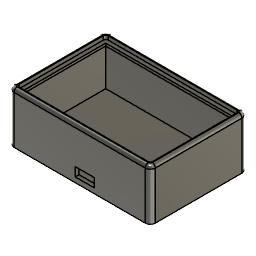
full macropad (Autodesk Fusion 360 archive; units mm, degrees)
design "macro  pad back up"
part number: 2026-03-02-20-18-01-878
Autodesk Fusion 360 part; units mm, degrees
sketch "Sketch1" plane through (0, 0, 0) normal (0, 0, 1) x (1, 0, 0)
  line L0 (-52.5, 35) -> (52.5, 35)
  line L1 (52.5, 35) -> (52.5, -35)
  line L2 (52.5, -35) -> (-52.5, -35)
  line L3 (-52.5, -35) -> (-52.5, 35)
  line L4 (-55.5, 38) -> (55.5, 38)
  line L5 (55.5, 38) -> (55.5, -38)
  line L6 (55.5, -38) -> (-55.5, -38)
  line L7 (-55.5, -38) -> (-55.5, 38)
  dimension "d1" = 105
  dimension "d2" = 70
  dimension "d3" = 35
  dimension "d4" = 52.5
  dimension "d5" = 111
  dimension "d6" = 76
  dimension "d7" = 3
  dimension "d8" = 3
  constraint horizontal L0
  constraint vertical L1
  constraint horizontal L2
  constraint vertical L3
  constraint horizontal L4
  constraint vertical L5
  constraint horizontal L6
  constraint vertical L7
  measures "d1" distance of L0.start L0.end
  measures "d2" distance of L0.start L2.end
  measures "d3" distance of origin L0
  measures "d4" distance of origin L3
  measures "d5" distance of L4.start L4.end
  measures "d6" distance of L4.start L6.end
  measures "d7" distance of L0 L4
  measures "d8" distance of L3 L7
extrude "Extrude1" add sketch "Sketch1" along normal blind 3 contours L0 L1 L2 L3 makes body 1
extrude "Extrude2" add sketch "Sketch1" along normal blind 40 bodies 1
fillet "Fillet1" radius 4 4 edges at (55.5, -38, 20) (55.5, 38, 20) (-55.5, -38, 20) (-55.5, 38, 20) on bodies 1
fillet "Fillet2" radius 2.5 8 edges at (54.3284, -36.8284, 40) (55.5, 0, 40) (54.3284, 36.8284, 40) (0, 38, 40) (-54.3284, 36.8284, 40) (-55.5, 0, 40) (-54.3284, -36.8284, 40) (0, -38, 40) on bodies 1
sketch "Sketch3" plane through (0, -38, 0) normal (0, -1, 0) x (1, 0, 0)
  line L0 (51.5, 37.5) -> (-51.5, 37.5)
  line L1 (-51.5, 37.5) -> (-51.5, 0)
  line L2 (-51.5, 0) -> (51.5, 0)
  line L3 (51.5, 0) -> (51.5, 37.5)
  line L4 (-3.5, 11) -> (11.5, 11)
  line L5 (11.5, 11) -> (11.5, 4)
  line L6 (11.5, 4) -> (-3.5, 4)
  line L7 (-3.5, 4) -> (-3.5, 11)
  dimension "d17" = 7
  dimension "d19" = 40
  dimension "d22" = 11
  dimension "d23" = 15
  constraint horizontal L4
  constraint vertical L5
  constraint horizontal L6
  constraint vertical L7
  measures "d17" distance of L4.start L6.end
  measures "d19" distance of L3 L5
  measures "d22" distance of L2 L4
  measures "d23" distance of L5 L7
extrude "Extrude3" cut sketch "Sketch3" against normal blind 10 contours L4 L5 L6 L7 bodies 1
sketch "Sketch5" plane through (0, 0, 40) normal (0, 0, 1) x (-1, 0, 0)
  line L0 (-52.5, 35) -> (52.5, 35)
  line L1 (52.5, 35) -> (52.5, -35)
  line L2 (52.5, -35) -> (-52.5, -35)
  line L3 (-52.5, -35) -> (-52.5, 35)
  arc A0 (-51.5, 35.5) -> (-53, 34) centre (-51.5, 34) ccw
  line L4 (-53, 34) -> (-53, -34)
  arc A1 (-53, -34) -> (-51.5, -35.5) centre (-51.5, -34) ccw
  line L5 (-51.5, -35.5) -> (51.5, -35.5)
  arc A2 (51.5, -35.5) -> (53, -34) centre (51.5, -34) ccw
  line L6 (53, -34) -> (53, 34)
  arc A3 (53, 34) -> (51.5, 35.5) centre (51.5, 34) ccw
  line L7 (51.5, 35.5) -> (-51.5, 35.5)
extrude "Extrude4" add sketch "Sketch5" against normal blind 2 separate body contours L0 L1 L2 L3 makes body 2
move_body "Move1" bodies 2 to x (1, 0, 0) y (0, 1, 0) z (0, 0, 1) at (0, 0, -3)
shell "Shell1" thickness 3 removed faces 2 at (17.5, -11.6667, 37) at (17.5, -11.6667, 35) on bodies 2
combine "Combine1" operation add target body 1 tool bodies 2
fillet "Fillet3" radius 2 4 edges at (-52.5, 35, 38.5) (-52.5, -35, 38.5) (52.5, -35, 38.5) (52.5, 35, 38.5) on bodies 1
